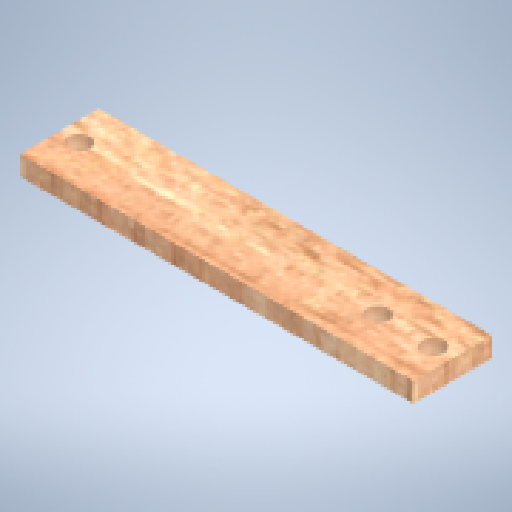
# Autodesk Inventor part: RollYAxis
Saved by Autodesk Inventor 2023 (Build 270158000, 158)
## iProperties
Created: 2023-10-26
Part Number: RollYAxis
Material: Wood (Birch)
Document SubType Name: Modeling
Designer: Mustapha
Density: 0.55 g/cm^3
Appearance: Birch - Natural Polished
Mass: 5.36933 g
Surface Area: 52.7775 cm^2
Volume: 9.76242 cm^3
Author: Mustapha
Autodesk Inventor part; units mm, degrees
ref_plane "YZ Plane" through (0, 0, 0) normal (1, 0, 0) x (0, 1, 0)
ref_plane "XZ Plane" through (0, 0, 0) normal (0, 1, 0) x (-1, 0, 0)
ref_plane "XY Plane" through (0, 0, 0) normal (0, 0, 1) x (1, 0, 0)
sketch "Sketch1" plane through (0, 0, 0) normal (0, 1, 0) x (-1, 0, 0)
  line L0 (0, 0) -> (100, 0)
  line L1 (100, 0) -> (100, -20)
  line L2 (100, -20) -> (0, -20)
  line L3 (0, -20) -> (0, 0)
  circle A0 centre (95, -10) radius 2.75
  circle A1 centre (5, -10) radius 2.75
  point P0 (0, -10)
  point P1 (100, -10)
  dimension "d0" = 20
  dimension "d1" = 100
  dimension "d2" = 5.5
  dimension "d3" = 5.5
  dimension "d4" = 5
  dimension "d5" = 5
  constraints: 8 end point, 2 centre point, 2 midpoint, 2 parallel, 1 horizontal, 1 perpendicular
  measures "d0" distance between parallel lines of L2 L0
  measures "d1" distance of L0.start L0.end
  measures "d2" diameter of A0
  measures "d3" diameter of A1
  measures "d4" distance of point (0, -10) A1.centre
  measures "d5" distance of A0.centre point (100, -10)
extrude "Extrusion1" add sketch "Sketch1" along normal blind 5
sketch "Sketch2" plane through (0, 0, 0) normal (0, -1, 0) x (1, 0, 0)
  circle A0 centre (-19.165, -10) radius 2.75
  circle A1 centre (-5, -10) radius 2.75 projected
  line L0 (-100, 0) -> (0, 0) projected
  dimension "d8" = 5.5
  dimension "d9" = 14.165
  dimension "d10" = 10
  constraints: 1 centre point
  measures "d8" diameter of A0
  measures "d9" distance of A0.centre A1.centre
  measures "d10" distance from line of L0 A0.centre
extrude "Extrusion2" cut sketch "Sketch2" against normal blind 10 contours A0
body "Solid1"
